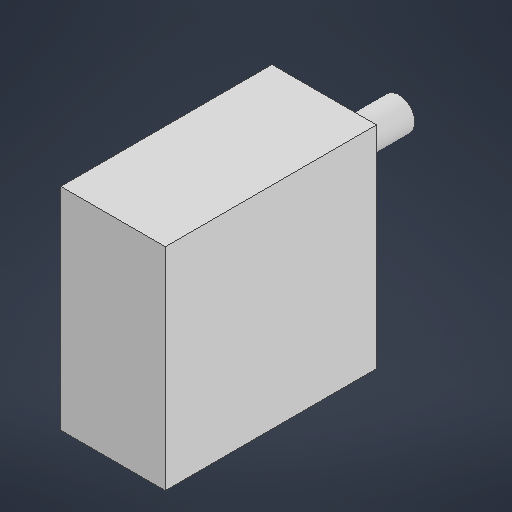
# Autodesk Inventor part: motor_basic
Saved by Autodesk Inventor 2026.2 (Build 302298000, 298)
## iProperties
Created: 2025-12-16
Part Number: motor_basic
Material: Generic
Document SubType Name: Modeling
Designer: Thoma
Density: 1 g/cm^3
Appearance: Default
Author: Thoma
Autodesk Inventor part; units mm, degrees
ref_plane "YZ Plane" through (0, 0, 0) normal (1, 0, 0) x (0, 1, 0)
ref_plane "XZ Plane" through (0, 0, 0) normal (0, 1, 0) x (-1, 0, 0)
ref_plane "XY Plane" through (0, 0, 0) normal (0, 0, 1) x (1, 0, 0)
sketch "Sketch1" plane through (0, 0, 0) normal (0, 0, 1) x (1, 0, 0)
  line L0 (4.16, 21.78) -> (23.76, 21.78)
  line L1 (23.76, 21.78) -> (23.76, -17.82)
  line L2 (23.76, -17.82) -> (4.16, -17.82)
  line L3 (4.16, -17.82) -> (4.16, 21.78)
  line L4 (4.16, 21.78) -> (23.76, 21.78)
  line L5 (13.96, 21.78) -> (13.96, 11.78)
  circle A0 centre (13.96, 11.78) radius 3
  point P0 (0, 0)
  dimension "d0" = 39.6
  dimension "d1" = 19.6
  dimension "d2" = 10
  dimension "d3" = 6
  constraints: 12 end point, 3 equal length, 1 centre point, 1 coincident, 1 horizontal, 1 midpoint, 1 perpendicular, 1 vertical
  measures "d0" distance of L0.end L1.end
  measures "d1" distance of L0.start L0.end
  measures "d2" distance of L5.start L5.end
  measures "d3" diameter of A0
extrude "Extrusion1" add sketch "Sketch1" along normal blind 39.6 contours L0 L1 L2 L3 | A0
sketch "Sketch2" plane through (0, 0, 0) normal (0, 0, -1) x (-1, 0, 0)
  line L0 (-23.76, 21.78) -> (-4.16, 21.78) projected
  line L1 (-23.76, 21.78) -> (-4.16, 21.78)
  line L2 (-13.96, 21.78) -> (-13.96, 11.78)
  circle A0 centre (-13.96, 11.78) radius 3
  point P0 (0, 0)
  dimension "d6" = 10
  dimension "d7" = 6
  constraints: 4 end point, 1 centre point, 1 coincident, 1 collinear, 1 midpoint, 1 vertical
  measures "d6" distance of L2.start L2.end
  measures "d7" diameter of A0
extrude "Extrusion2" add sketch "Sketch2" along normal blind 10
sketch "Sketch3" plane through (13.96, 11.78, -10) normal (0, 0, -1) x (-1, 0, 0)
  circle A0 centre (0, 0) radius 3 projected
  circle A1 centre (0, 0) radius 3
  point P0 (13.96, -11.78)
  constraints: 1 centre point, 1 coincident
extrude "Extrusion3" add sketch "Sketch3" along normal blind 4
body "Solid1"
